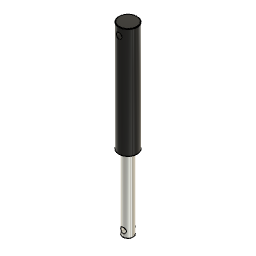
pick up truck v26 (Autodesk Fusion 360 archive; units mm, degrees)
design "Actuator"
Autodesk Fusion 360 part; units mm, degrees
sketch "Sketch1" plane through (0, 0, 0) normal (0, 0, 1) x (1, 0, 0)
  circle A0 centre (0, 0) radius 50
  line L0 (36, 0) -> (36, 6)
  line L1 (36, 6) -> (29.3939, 6)
  line L2 (36, 0) -> (36, -6)
  line L3 (36, -6) -> (29.3939, -6)
  arc A1 (29.3939, 6) -> (29.3939, -6) centre (0, 0) ccw
  dimension "d1" = 100
  dimension "d2" = 60
  dimension "d3" = 36
  dimension "d4" = 6
  dimension "d5" = 6
  constraint coincident A0.centre A1.centre
  constraint perpendicular L0 L1
  constraint perpendicular L0 L3
  measures "d1" diameter of A0
  measures "d2" diameter of A1
  measures "d3" distance of A0.centre L0.start
  measures "d4" distance of L0.start L0.end
  measures "d5" distance of L0.start L2.end
extrude "Extrude1" add sketch "Sketch1" against normal blind 600 makes body 1
extrude "Extrude2" add sketch "Sketch1" against normal blind 100 contours L0 L1 L2 L3 A1 bodies 1
sketch "Sketch2" plane through (0, 0, -600) normal (0, 0, -1) x (1, 0, 0)
  line L0 (36, 6) -> (36, -6)
  line L1 (36, -6) -> (29.3939, -6)
  arc A0 (29.3939, 6) -> (29.3939, -6) centre (0, 0) ccw
  line L2 (29.3939, 6) -> (36, 6)
  circle A1 centre (0, 0) radius 50
  line L3 (36, -6) -> (36, 6)
  line L4 (36, 6) -> (29.3939, 6)
  arc A2 (29.3939, 6) -> (29.3939, -6) centre (0, 0) ccw
  line L5 (29.3939, -6) -> (36, -6)
  line L6 (34, -4) -> (27.7128, -4)
  arc A3 (27.7128, 4) -> (27.7128, -4) centre (0, 0) ccw
  line L7 (27.7128, 4) -> (34, 4)
  line L8 (34, 4) -> (34, -4)
  dimension "d10" = -2
extrude "Extrude3" add sketch "Sketch2" along normal blind 400 and the other way blind 50 separate body contours L6 A3 L7 L8 makes body 2
sketch "Sketch3" plane through (0, 0, -1000) normal (0, 0, -1) x (1, 0, 0)
  arc A0 (27.7128, 4) -> (27.7128, -4) centre (0, 0) ccw
  line L0 (27.7128, -4) -> (34, -4)
  line L1 (34, -4) -> (34, 4)
  line L2 (34, 4) -> (27.7128, 4)
  circle A1 centre (0, 0) radius 28
  constraint concentric A0 A1
extrude "Extrude4" cut sketch "Sketch3" against normal blind 405 contours L0 L1 L2 A1 bodies 2
copy_body "Body->Comp1" bodies 2 removing the originals makes body 3 in component "Shaft"
fillet "Fillet1" radius 2.5 1 edges at (-46.6164, -18.0808, 0) on bodies 1
fillet "Fillet2" radius 2.5 1 edges at (-46.6164, 18.0808, -600) on bodies 1
fillet "Fillet1'" radius 2.5 1 edges at (-24.391, 13.7507, -1000) on bodies 3 in component "Shaft"
hole "Hole1" at (0, 28, -966.109) direction (0, -1, 0) diameter 30 depth 100 tip angle 118 bodies 3 in component "Shaft"
hole "Hole1'" at (0, 50, -41.9196) direction (0, -1, 0) diameter 30 depth 100 tip angle 118 bodies 1
component "Shaft" placed x (1, 0, 0) y (0, 1, 0) z (0, 0, 1) at (0, 0, 0)
